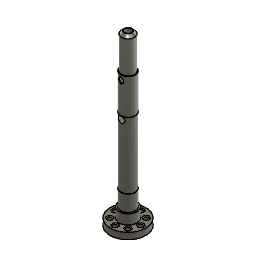
Task1 v4 (Autodesk Fusion 360 design; units mm, degrees)
Autodesk Fusion 360 part; units mm, degrees
sketch "Sketch1" plane through (0, 0, 0) normal (0, 1, 0) x (1, 0, 0)
  circle A0 centre (0, 0) radius 11
  dimension "d1" = 22
  constraint coincident A0.centre origin
  measures "d1" diameter of A0
extrude "Extrude1" add sketch "Sketch1" along normal blind 4
sketch "Sketch2" plane through (0, 4, 0) normal (0, 1, 0) x (-1, 0, 0)
  circle A0 centre (0, 0) radius 11
  circle A1 centre (0, 0) radius 8 construction
  circle A2 centre (0, -8) radius 1.35
  line L0 (0, -8) -> (0, 0)
  circle A3 centre (5.6569, -5.6569) radius 1.35
  circle A4 centre (8, 0) radius 1.35
  circle A5 centre (5.6569, 5.6569) radius 1.35
  circle A6 centre (0, 8) radius 1.35
  circle A7 centre (-5.6569, 5.6569) radius 1.35
  circle A8 centre (-8, 0) radius 1.35
  circle A9 centre (-5.6569, -5.6569) radius 1.35
  dimension "d4" = 16
  dimension "d5" = 2.7
  dimension "d7" = 360
  constraint coincident A0.centre A1.centre
  constraint coincident A1 A2.centre
  constraint coincident A2.centre L0.start
  constraint vertical L0
  measures "d4" diameter of A1
  measures "d5" diameter of A2
hole "Hole1" at (-5.6569, 4, -5.6569) at (-8, 4, 0) at (-5.6569, 4, 5.6569) at (0, 4, 8) at (5.6569, 4, 5.6569) at (8, 4, 0) at (5.6569, 4, -5.6569) at (0, 4, -8) direction (0, -1, 0) diameter 2.7 depth 5 tip angle 180 countersink diameter 3.7 countersink angle 90
sketch "Sketch3" plane through (0, 4, 0) normal (0, 1, 0) x (-1, 0, 0)
  circle A0 centre (-5.6569, -5.6569) radius 1.85
  circle A1 centre (-5.6569, 5.6569) radius 1.85
  circle A2 centre (5.6569, 5.6569) radius 1.85
  circle A3 centre (5.6569, -5.6569) radius 1.85
  circle A4 centre (8, 0) radius 1.85
  circle A5 centre (0, 8) radius 1.85
  circle A6 centre (-8, 0) radius 1.85
  circle A7 centre (0, -8) radius 1.85
  circle A8 centre (0, 0) radius 11
  circle A9 centre (0, 0) radius 5.5
  dimension "d13" = 11
  constraint concentric A8 A9
  measures "d13" diameter of A9
extrude "Extrude2" add sketch "Sketch3" along normal blind 6 contours A9
sketch "Sketch4" plane through (0, 0, 0) normal (0, -1, 0) x (1, 0, 0)
  circle A0 centre (5.6569, -5.6569) radius 1.35
  circle A1 centre (5.6569, 5.6569) radius 1.35
  circle A2 centre (-5.6569, 5.6569) radius 1.35
  circle A3 centre (-5.6569, -5.6569) radius 1.35
  circle A4 centre (-8, 0) radius 1.35
  circle A5 centre (0, 8) radius 1.35
  circle A6 centre (8, 0) radius 1.35
  circle A7 centre (0, -8) radius 1.35
  circle A8 centre (0, 0) radius 11
  circle A9 centre (0, 0) radius 4
  dimension "d16" = 8
  constraint coincident A8.centre A9.centre
  measures "d16" diameter of A9
hole "Hole2" at (0, 0, 0) direction (0, 1, 0) diameter 8 depth 7.3 tip angle 118
sketch "Sketch5" plane through (0, 10, 0) normal (0, 1, 0) x (-1, 0, 0)
  circle A0 centre (0, 0) radius 5.5
  circle A1 centre (0, 0) radius 4.5
  dimension "d20" = 9
  constraint concentric A0 A1
  measures "d20" diameter of A1
extrude "Extrude3" add sketch "Sketch5" along normal blind 10 contours A1
sketch "Sketch6" plane through (0, 20, 0) normal (0, 1, 0) x (-1, 0, 0)
  circle A0 centre (0, 0) radius 4.5
  circle A1 centre (0, 0) radius 4.4
  dimension "d23" = 8.8
  constraint concentric A0 A1
  measures "d23" diameter of A1
extrude "Extrude4" add sketch "Sketch6" along normal blind 41 contours A1
sketch "Sketch7" plane through (0, 61, 0) normal (0, 1, 0) x (-1, 0, 0)
  circle A0 centre (0, 0) radius 4.4
  circle A1 centre (0, 0) radius 4.5
  dimension "d26" = 9
  constraint concentric A0 A1
  measures "d26" diameter of A1
extrude "Extrude5" add sketch "Sketch7" along normal blind 22 contours A0 | A1
sketch "Sketch8" plane through (0, 83, 0) normal (0, 1, 0) x (-1, 0, 0)
  circle A0 centre (0, 0) radius 4.5
  circle A1 centre (0, 0) radius 4
  dimension "d29" = 8
  constraint coincident A0.centre A1.centre
  measures "d29" diameter of A1
extrude "Extrude6" add sketch "Sketch8" along normal blind 21.5 contours A1
chamfer "Chamfer1" distance 1.6 angle 45 1 edges at (3.7293, 104.5, -1.4465)
ref_plane "WorkPlane1" through (0, 0, 4.5) normal (0, 0, 1) x (1, 0, 0)
sketch "Sketch9" plane through (0, 0, 4.5) normal (0, 0, 1) x (1, 0, 0)
  line L0 (-2.4, 104.5) -> (2.4, 104.5)
  circle A0 centre (0, 59) radius 2
  line L1 (0, 0) -> (0, 59) construction
  circle A1 centre (0, 80) radius 1.25
  line L2 (0, 59) -> (0, 80) construction
  dimension "d34" = 4
  dimension "d35" = 45.5
  dimension "d36" = 2.5
  dimension "d37" = 24.5
  constraint coincident L1.start origin
  constraint coincident A0.centre L1.end
  constraint vertical L1
  constraint coincident A1.centre L2.end
  constraint vertical L2
  measures "d34" diameter of A0
  measures "d35" distance of L0 A0.centre
  measures "d36" diameter of A1
  measures "d37" distance of L0 A1.centre
hole "Hole3" at (0, 80, 4.5) direction (0, 0, -1) diameter 2.5 depth 4.5 tip angle 118 countersink diameter 3.5 countersink angle 90
extrude "Extrude7" cut sketch "Sketch9" against normal blind 4.5 contours A0
sketch "Sketch10" plane through (0, 104.5, 0) normal (0, 1, 0) x (-1, 0, 0)
  circle A0 centre (0, 0) radius 2.4
  circle A1 centre (0, 0) radius 2
  dimension "d45" = 4
  constraint concentric A0 A1
  measures "d45" diameter of A1
extrude "Extrude8" cut sketch "Sketch10" against normal blind 45.5 contours A1
chamfer "Chamfer2" distance 0.1 angle 45 1 edges at (4.1955, 20, -1.6273) measured on face at (1.8338, 20, -4.0606)
chamfer "Chamfer3" distance 0.1 angle 45 1 edges at (4.1955, 61, -1.6273) measured on face at (1.8935, 74.6224, 4.0822)
chamfer "Chamfer4" distance 1.9999 angle 45 1 edges at (0, 59, 0) measured on face at (-0.4778, 57.6498, 0)
